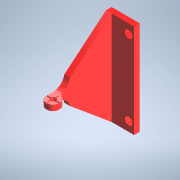
# Autodesk Inventor part: camera_holder
Saved by Autodesk Inventor 2022 (Build 260153000, 153)
## iProperties
Created: 2022-10-11
Part Number: camera_holder
Material: Типовые
Document SubType Name: Modeling
Designer: korsh624
Density: 1 g/cm^3
Appearance: Светло-красный
Author: korsh624
Autodesk Inventor part; units mm, degrees
ref_plane "YZ Plane" through (0, 0, 0) normal (1, 0, 0) x (0, 1, 0)
ref_plane "XZ Plane" through (0, 0, 0) normal (0, 1, 0) x (-1, 0, 0)
ref_plane "XY Plane" through (0, 0, 0) normal (0, 0, 1) x (1, 0, 0)
sketch "Эскиз1" plane through (0, 0, 0) normal (0, 0, 1) x (1, 0, 0)
  circle A0 centre (-65.4674, -23.2) radius 2 projected
  circle A1 centre (-65.4674, -63.2) radius 2 projected
  line L0 (-62.5517, -18.2) -> (-77.5517, -18.2)
  line L1 (-77.5517, -18.2) -> (-77.5517, -68.2)
  line L2 (-77.5517, -68.2) -> (-62.5517, -68.2)
  line L3 (-62.5517, -68.2) -> (-62.5517, -18.2)
  point P0 (0, 0)
  dimension "d0" = 15
  dimension "d1" = 50
  dimension "d2" = 40
  dimension "d3" = 5
  constraints: 8 end point, 2 parallel, 1 horizontal, 1 perpendicular
  measures "d0" distance of L2.end L1.end
  measures "d1" distance of L1.end L0.end
  measures "d2" distance of A1.centre A0.centre
  measures "d3" distance from line of A1.centre L2
extrude "Выдавливание1" add sketch "Эскиз1" along normal blind 3
sketch "Эскиз2" plane through (-77.5517, -68.2, 0) normal (-1, 0, 0) x (0, 0, 1)
  line L0 (3, 50) -> (3, 0) projected
  line L1 (3, 25) -> (38, 25) construction
  line L2 (3, 50) -> (33, 25)
  line L3 (31.2, 23.5) -> (3, 0)
  line L4 (38, 26.5) -> (31.2, 26.5)
  line L5 (31.2, 23.5) -> (38, 23.5)
  line L6 (38, 23.5) -> (38, 26.5)
  point P0 (0, 68.2)
  dimension "d6" = 35
  dimension "d7" = 30
  dimension "d8" = 1.5
  dimension "d9" = 1.5
  constraints: 12 end point, 2 horizontal, 2 point on line, 1 midpoint, 1 parallel
  measures "d6" distance of L1.start L1.end
  measures "d7" distance of L2.end L1.start
  measures "d8" distance between parallel lines of L4 L1
  measures "d9" distance between parallel lines of L5 L1
extrude "Выдавливание2" add sketch "Эскиз2" against normal blind 3
sketch "Эскиз3" plane through (-77.5517, -41.7, 38) normal (0, 1, 0) x (1, 0, 0)
  line L0 (0, 0) -> (0, 6.8) projected
  line L1 (0, 0) -> (3, 0) projected
  line L2 (0, 6.8) -> (3, 6.8) projected
  line L3 (0, 6.8) -> (6.8, 6.8)
  line L4 (6.8, 6.8) -> (6.8, 0)
  line L5 (6.8, 0) -> (0, 0)
  line L6 (0, 0) -> (0, 6.8)
  line L7 (3, 6.8) -> (3, 0) projected
  point P0 (77.5517, 38)
  dimension "d12" = 3
  dimension "d13" = 3.8
  dimension "d14" = 6.8
  constraints: 8 end point, 2 parallel, 1 horizontal, 1 perpendicular
  measures "d12" distance between parallel lines of L0 L7
  measures "d13" distance between parallel lines of L4 L7
  measures "d14" distance of L3.end L4.end
extrude "Выдавливание3" add sketch "Эскиз3" against normal blind 3 contours L7 L3 L4 L5
fillet "Сопряжение1" radius 3 3 edges at (-77.5517, -43.2, 38) (-70.7517, -43.2, 38) (-70.7517, -43.2, 31.2)
fillet "Сопряжение2" radius 3 1 edges at (-74.5517, -43.2, 31.2)
sketch "Эскиз4" plane through (-77.5517, -41.7, 31.2) normal (0, 1, 0) x (1, 0, 0)
  line L0 (0, 0) -> (3, 0) projected
  line L1 (0, -3.8) -> (0, 0) projected
  arc A0 (0, -3.8) -> (3, -6.8) centre (3, -3.8) ccw projected
  line L2 (3, -6.8) -> (3.8, -6.8) projected
  arc A1 (3.8, -6.8) -> (6.8, -3.8) centre (3.8, -3.8) ccw projected
  line L3 (6.8, -3.8) -> (6.8, -3) projected
  arc A2 (6.8, -3) -> (4.9, -0.2089) centre (3.8, -3) ccw projected
  arc A3 (3, 2.5821) -> (4.9, -0.2089) centre (6, 2.5821) ccw projected
  line L4 (3, 0) -> (3, 2.5821) projected
  circle A4 centre (3.4, -3.4) radius 1.5
  point P0 (77.5517, 31.2)
  dimension "d19" = 3
  constraints: 1 centre point
  measures "d19" diameter of A4
extrude "Выдавливание4" cut sketch "Эскиз4" against normal blind 3 contours A4
sketch "Эскиз5" plane through (-77.5517, -41.7, 31.2) normal (0, 1, 0) x (1, 0, 0)
  circle A0 centre (3.4, -3.4) radius 1.5 projected
  line L0 (3.5681, -7.5363) -> (3.1342, -7.5363)
  line L1 (3.1342, -7.5363) -> (3.1342, -0.5127)
  line L2 (3.1342, -0.5127) -> (3.5681, -0.5127)
  line L3 (3.5681, -0.5127) -> (3.5681, -7.5363)
  line L4 (7.324, -3.794) -> (-1.1504, -3.794)
  line L5 (-1.1504, -3.794) -> (-1.1504, -3.1974)
  line L6 (-1.1504, -3.1974) -> (7.324, -3.1974)
  line L7 (7.324, -3.1974) -> (7.324, -3.794)
  point P0 (77.5517, 31.2)
  point P1 (1.9527, -3.794)
  point P2 (1.9137, -3.1974)
  point P3 (4.8863, -3.1974)
  point P4 (4.8473, -3.794)
  point P5 (3.1342, -1.9237)
  point P6 (3.5681, -1.9095)
  point P7 (3.5681, -4.8905)
  point P8 (3.1342, -4.8763)
  constraints: 16 end point, 4 parallel, 2 horizontal, 2 perpendicular
extrude "Выдавливание5" cut sketch "Эскиз5" against normal blind 0.5 contours A0 L6 L7 L4 | A0 L1 L2 L3 | L3 L0 L1 A0 | A0 L4 L5 L6
sketch "Эскиз6" plane through (-77.5517, -68.2, 0) normal (-1, 0, 0) x (0, 0, 1)
  line L0 (34.3974, 26.5) -> (31.2, 26.5) projected
  line L1 (31.2, 23.5) -> (35, 23.5) projected
  line L2 (31.2, 26.5) -> (28.6179, 26.5) projected
  line L3 (31.2, 26.5) -> (25.2, 26.5)
  line L4 (25.2, 26.5) -> (25.2, 31.9489)
  line L5 (25.2, 31.9489) -> (31.2, 31.9489)
  line L6 (31.2, 26.5) -> (3, 50) projected
  line L7 (31.2, 31.9489) -> (31.2, 26.5)
  line L8 (31.2, 23.5) -> (25.2, 23.5)
  line L9 (25.2, 23.5) -> (25.2, 16.2347)
  line L10 (25.2, 16.2347) -> (31.2, 23.5)
  point P0 (0, 68.2)
  point P1 (25.2, 31.5)
  dimension "d24" = 6
  constraints: 14 end point, 4 perpendicular, 1 collinear, 1 horizontal
  measures "d24" distance of L0.end L3.end
extrude "Выдавливание6" cut sketch "Эскиз6" against normal blind 3 contours L2 L3 L4 L6 | L10 L9 L8
fillet "Сопряжение3" radius 6 2 edges at (-76.0517, -41.7, 25.2) (-76.0517, -44.7, 25.2)
